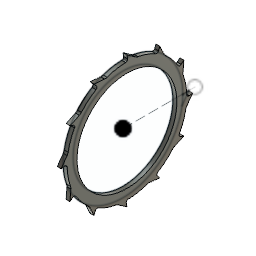
Unidirectional Cleat with Parameters (Autodesk Fusion 360 design; units mm, degrees)
Autodesk Fusion 360 part; units mm, degrees
sketch "Sketch1" plane through (0, 0, 0) normal (1, 0, 0) x (0, 1, 0)
  circle A0 centre (0, 0) radius 25
  circle A1 centre (0, 0) radius 30
  line L0 (0, 0) -> (30, 0) construction
  line L1 (30, 0) -> (33, 0) construction
  line L2 (33, 0) -> (29.9953, -0.5298)
  line L3 (33, 0) -> (36.051, 0) construction
  line L4 (33, 0) -> (29.6058, -4.8474)
  dimension "d7" = 50
  dimension "d8" = 60
  dimension "d10" = 3
  dimension "d11" = 170
  dimension "d12" = 135
  constraint coincident A0.centre A1.centre
  constraint concentric A0 A1
  constraint coincident A1 L0.end
  constraint horizontal L0
  constraint parallel L0 L1
  constraint horizontal L3
  constraint coincident A1 L2.end
  constraint coincident A1 L4.end
  measures "d7" diameter of A0
  measures "d8" diameter of A1
  measures "d10" distance of L0.end L1.end
  measures "d11" angle of L2 L3
  measures "d12" angle of L2 L4
extrude "Extrude1" add sketch "Sketch1" along normal blind 2 contours A1
extrude "Extrude2" add sketch "Sketch1" along normal blind 2 contours A1 L2 L4
fillet "Fillet1" radius 1 1 edges at (1, 29.9953, -0.5298)
fillet "Fillet2" radius 3 1 edges at (1, 29.6058, -4.8474)
pattern_circular "C-Pattern1" count 12 over 360 about axis through (1.75, 0, 0) along (1, 0, 0) of "Extrude2", "Fillet1", "Fillet2"
equation "inner_diameter = 50 mm"
equation "outer_diameter = 60 mm"
equation "spike_length = 3 mm"
equation "spikes = 12"
equation "rake = 10 deg"
equation "relief = 45 deg"
equation "d7 = inner_diameter"
equation "d8 = outer_diameter"
equation "d10 = spike_length"
equation "d11 = 180 deg - rake"
equation "d12 = 180 deg - relief"
equation "thickness = 2 mm"
equation "d14 = thickness"
equation "rake_fillet = 1 mm"
equation "relief_fillet = 3 mm"
equation "d21 = rake_fillet"
equation "d23 = relief_fillet"
equation "d24 = spikes"
